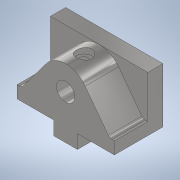
# Autodesk Inventor part: Pieza4_corredera_LAASR
Saved by Autodesk Inventor 2021 (Build 250183000, 183)
## iProperties
Created: 2020-10-13
Part Number: Pieza4_corredera_LAASR
Material: Steel, Carbon
Document SubType Name: Modeling
Designer: CASA
Density: 7.85 g/cm^3
Appearance: Semi-Polished
Author: CASA
Autodesk Inventor part; units mm, degrees
ref_plane "YZ Plane" through (0, 0, 0) normal (1, 0, 0) x (0, 1, 0)
ref_plane "XZ Plane" through (0, 0, 0) normal (0, 1, 0) x (-1, 0, 0)
ref_plane "XY Plane" through (0, 0, 0) normal (0, 0, 1) x (1, 0, 0)
sketch "Sketch1" plane through (0, 0, 0) normal (0, 0, 1) x (1, 0, 0)
  line L0 (-32, 23) -> (32, 23)
  line L1 (32, 23) -> (32, -13)
  line L2 (7.75, -23) -> (-7.75, -23)
  line L3 (-32, -13) -> (-32, 23)
  line L4 (7.75, -13) -> (32, -13)
  line L5 (7.75, -23) -> (7.75, -13)
  line L6 (-32, -13) -> (-7.75, -13)
  line L7 (-7.75, -13) -> (-7.75, -23)
  point P0 (0, 0)
  dimension "d2" = 32
  dimension "d3" = 23
  constraints: 16 end point, 3 horizontal, 2 parallel, 2 perpendicular
  measures "d2" distance from line of L1 point (0, 0)
  measures "d3" distance from line of L0 point (0, 0)
extrude "Extrusion1" add sketch "Sketch1" along normal blind 10
sketch "Sketch2" plane through (0, 0, 10) normal (0, 0, 1) x (1, 0, 0)
  line L0 (-32, -13) -> (-7.75, -13) projected
  line L1 (-32, -13) -> (-32, -5)
  line L2 (-32, 23) -> (-32, -13) projected
  line L3 (-32, -5) -> (-29, -5)
  line L4 (32, -13) -> (32, 23) projected
  line L5 (32, -9) -> (32, -5)
  line L6 (32, -5) -> (29, -5)
  line L7 (-7.75, -13) -> (-7.75, -23) projected
  line L8 (7.75, -13) -> (32, -13) projected
  arc A0 (12.8, 16.6) -> (-12.8, 16.6) centre (0, 7) ccw
  line L9 (-29, -5) -> (-12.8, 16.6)
  line L10 (29, -5) -> (12.8, 16.6)
  line L11 (-32, -13) -> (-7.75, -13)
  line L12 (-7.75, -23) -> (7.75, -23) projected
  line L13 (-7.75, -23) -> (7.75, -23)
  line L14 (7.75, -23) -> (7.75, -13) projected
  line L15 (7.75, -23) -> (7.75, -13)
  line L16 (7.75, -13) -> (32, -13)
  line L17 (32, -5) -> (32, -13)
  point P0 (0, 0)
  dimension "d15" = 32
  constraints: 22 end point, 4 collinear, 3 point on line, 2 horizontal, 2 point on circle, 2 tangent, 1 centre point, 1 perpendicular
  measures "d15" diameter of A0
extrude "Extrusion2" add sketch "Sketch2" along normal blind 22
sketch "Sketch3" plane through (0, 0, 32) normal (0, 0, 1) x (1, 0, 0)
  line L0 (-32, -5) -> (-32, -13) projected
  circle A0 centre (0, 7) radius 6
  point P0 (0, 0)
  constraints: 1 centre point
extrude "Extrusion3" cut sketch "Sketch3" against normal through all
sketch "Sketch5" plane through (-32, 23, 0) normal (0, 1, 0) x (1, 0, 0)
  line L0 (32, 0) -> (32, -20)
  circle A0 centre (32, -20) radius 5
  circle A1 centre (32, -20) radius 2.875
  dimension "d22" = 20
  dimension "d23" = 10
  dimension "d36" = 5.75
  constraints: 2 centre point, 2 coincident, 2 end point, 1 vertical
  measures "d22" distance of L0.start L0.end
  measures "d23" diameter of A0
  measures "d36" diameter of A1
extrude "Extrusion4" cut sketch "Sketch5" against normal blind 12 contours A1
extrude "Extrusion5" cut sketch "Sketch5" against normal blind 4 contours A0 | A1
sketch "Sketch6" plane through (-7.75, -23, 0) normal (0, -1, 0) x (1, 0, 0)
  point P0 (7.75, 0)
sketch "Sketch7" plane through (-7.75, -23, 0) normal (0, -1, 0) x (1, 0, 0)
  line L0 (0, 32) -> (15.5, 32) projected
  circle A0 centre (7.75, 24) radius 3
  circle A1 centre (7.75, 8) radius 3
  point P0 (7.75, 0)
  dimension "d31" = 6
  dimension "d32" = 6
  constraints: 2 centre point
  measures "d31" diameter of A0
  measures "d32" diameter of A1
extrude "Extrusion6" cut sketch "Sketch7" against normal blind 18
fillet "Fillet1" radius 3 2 edges at (29, -5, 21) (-29, -5, 21)
sketch "Sketch8" plane through (0, 0, 32) normal (0, 0, 1) x (1, 0, 0)
  line L0 (-7.75, -22) -> (7.75, -22)
  line L1 (7.75, -22) -> (7.75, -23)
  line L2 (7.75, -23) -> (-7.75, -23)
  line L3 (-7.75, -23) -> (-7.75, -22)
  line L4 (-7.75, -23) -> (7.75, -23) projected
  line L5 (-7.75, -13) -> (-7.75, -23) projected
  line L6 (7.75, -23) -> (7.75, -13) projected
  point P0 (0, 0)
  dimension "d37" = 1
  constraints: 8 end point, 3 collinear, 2 parallel, 1 horizontal, 1 perpendicular
  measures "d37" distance of L0.end L1.end
extrude "Extrusion7" cut sketch "Sketch8" against normal through all
body "Solid1"
